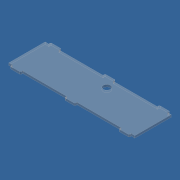
# Autodesk Inventor part: P1704_003
Saved by Autodesk Inventor 2015 (Build 190159000, 159)
## iProperties
Created: 2017-02-08
Part Number: P1704_003
Project: Polymanette chevalier
Material: Plastique PMMA
Description: Paroi avant
Document SubType Name: Modeling
Designer: Alexandre.PICOTTE
Authority: 180x58x3
Density: 1.188 g/cm^3
Appearance: Transparent - Clair
Mass: 33.9948 g
Surface Area: 206.988 cm^2
Volume: 28.6152 cm^3
Material number: ---
Author: Boris.GAUDARD
Autodesk Inventor part; units mm, degrees
ref_plane "Plan YZ" through (0, 0, 0) normal (1, 0, 0) x (0, 1, 0)
ref_plane "Plan XZ" through (0, 0, 0) normal (0, 1, 0) x (-1, 0, 0)
ref_plane "Plan XY" through (0, 0, 0) normal (0, 0, 1) x (1, 0, 0)
sketch "Esquisse12" plane through (0, 0, 0) normal (0, 0, 1) x (1, 0, 0)
  line L0 (-90, -26) -> (-90, 26)
  line L1 (-90, 26) -> (-85, 26)
  line L2 (-85, 26) -> (-85, 29)
  line L3 (-85, 29) -> (-70, 29)
  line L4 (-70, 29) -> (-70, 26)
  line L5 (7.5, 26) -> (7.5, 29)
  line L6 (7.5, 29) -> (-7.5, 29)
  line L7 (-7.5, 29) -> (-7.5, 26)
  line L8 (70, 26) -> (70, 29)
  line L9 (70, 29) -> (85, 29)
  line L10 (85, 29) -> (85, 26)
  line L11 (85, 26) -> (90, 26)
  line L12 (90, 26) -> (90, -26)
  line L13 (90, -26) -> (85, -26)
  line L14 (85, -26) -> (85, -29)
  line L15 (85, -29) -> (70, -29)
  line L16 (70, -29) -> (70, -26)
  line L17 (-7.5, -26) -> (-7.5, -29)
  line L18 (7.5, -29) -> (7.5, -26)
  line L19 (-70, -26) -> (-70, -29)
  line L20 (-85, -29) -> (-85, -26)
  line L21 (-90, -26) -> (-85, -26)
  line L22 (-85, -29) -> (-70, -29)
  line L23 (7.5, -29) -> (-7.5, -29)
  line L24 (-70, 26) -> (-7.5, 26)
  line L25 (7.5, 26) -> (70, 26)
  line L26 (7.5, -26) -> (70, -26)
  line L27 (-7.5, -26) -> (-70, -26)
  line L28 (-126, 0) -> (126, 0) projected
  line L29 (0, -40.6) -> (0, 40.6) projected
  point P0 (0, 0)
  dimension "d86" = 52
  dimension "d87" = 3
  dimension "d88" = 5
  dimension "d90" = 15
  dimension "d106" = 77.5
  constraints: 56 end point, 27 point on line, 10 perpendicular, 7 equal length, 3 collinear, 2 parallel, 2 vertical, 1 horizontal, 2 other
  measures "d86" distance of L0.start L0.end
  measures "d87" distance of L1.end L2.end
  measures "d88" distance of L0.end L1.end
  measures "d90" distance of L2.end L3.end
  measures "d106" distance between parallel lines of L7 L2
extrude "Extrusion5" add sketch "Esquisse12" along normal blind 3
sketch "Esquisse13" plane through (0, 0, 3) normal (0, 0, 1) x (1, 0, 0)
  point P0 (0, 0)
  point P1 (-85, 26)
  point P2 (-70, 26)
  point P3 (-85, -26)
  point P4 (-70, -26)
  point P5 (-7.5, -26)
  point P6 (7.5, -26)
  point P7 (70, -26)
  point P8 (85, -26)
  point P9 (85, 26)
  point P10 (70, 26)
  point P11 (-7.5, 26)
  point P12 (7.5, 26)
hole "Perçage6" at (-85, 26, 3) at (-70, 26, 3) at (-85, -26, 3) at (-70, -26, 3) at (-7.5, -26, 3) at (7.5, -26, 3) at (70, -26, 3) at (85, -26, 3) at (85, 26, 3) at (70, 26, 3) at (-7.5, 26, 3) at (7.5, 26, 3) direction (0, 0, -1) diameter 1 end through all
chamfer "Chanfrein3" distance 1 angle 45 12 edges at (-85, 29, 1.5) (-70, 29, 1.5) (-7.5, 29, 1.5) (7.5, 29, 1.5) (70, 29, 1.5) (85, 29, 1.5) (-85, -29, 1.5) (-70, -29, 1.5) (-7.5, -29, 1.5) (7.5, -29, 1.5) (70, -29, 1.5) (85, -29, 1.5)
sketch "Esquisse14" plane through (0, 0, 3) normal (0, 0, 1) x (1, 0, 0)
  circle A0 centre (10.2, 13.8) radius 5
  line L0 (-90, 26) -> (-90, -26) projected
  line L1 (8, -26) -> (69.5, -26) projected
  point P0 (0, 0)
  dimension "d107" = 100.2
  dimension "d108" = 39.8
  dimension "d109" = 10
  constraints: 1 centre point
  measures "d107" distance from line of L0 A0.centre
  measures "d108" distance from line of L1 A0.centre
  measures "d109" diameter of A0
extrude "Extrusion6" cut sketch "Esquisse14" against normal through all
